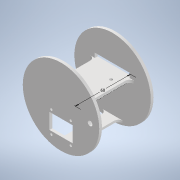
# Autodesk Inventor part: top2
Saved by Autodesk Inventor 2022 (Build 260153000, 153)
## iProperties
Created: 2025-06-18
Part Number: top2
Material: Типовые
Document SubType Name: Modeling
Designer: korsh624
Density: 1 g/cm^3
Appearance: По умолчанию
Author: korsh624
Autodesk Inventor part; units mm, degrees
ref_plane "YZ Plane" through (0, 0, 0) normal (1, 0, 0) x (0, 1, 0)
ref_plane "XZ Plane" through (0, 0, 0) normal (0, 1, 0) x (-1, 0, 0)
ref_plane "XY Plane" through (0, 0, 0) normal (0, 0, 1) x (1, 0, 0)
sketch "Эскиз3" plane through (0, 0, 0) normal (0, 0, 1) x (1, 0, 0)
  circle A0 centre (0, 0) radius 41.5
  line L0 (12.5, -11.0597) -> (-12.5, -11.0597) projected
  line L1 (-12.5, -11.0597) -> (-12.5, -28.0597) projected
  line L2 (-12.5, -11.0597) -> (12.5, -11.0597)
  line L3 (12.5, -11.0597) -> (12.5, -28.0597)
  line L4 (12.5, -28.0597) -> (-12.5, -28.0597)
  line L5 (-12.5, -28.0597) -> (-12.5, -11.0597)
  dimension "d9" = 83
  dimension "d10" = 25
  dimension "d11" = 17
  dimension "d13" = 25
  dimension "d14" = 17
  dimension "d15" = 12.5
  constraints: 8 end point, 2 parallel, 1 centre point, 1 coincident, 1 horizontal, 1 perpendicular
  measures "d9" diameter of A0
  measures "d10" distance of L0.start L0.end
  measures "d11" distance of L0.end L1.end
  measures "d13" distance of L2.start L2.end
  measures "d14" distance of L2.end L3.end
  measures "d15" distance from line of point (0, 0) L5
extrude "Выдавливание3" add sketch "Эскиз3" along normal blind 3
sketch "Эскиз4" plane through (0, 0, 3) normal (0, 0, 1) x (1, 0, 0)
  arc A0 (5.7629, -8.6636) -> (-4.709, -8.7124) centre (0.4132, 15.7598) ccw
  circle A1 centre (0.4132, 15.7598) radius 1.5338
  point P0 (0, 0)
  constraints: 2 centre point, 2 point on circle, 1 coincident, 4 other
extrude "Выдавливание4" cut sketch "Эскиз4" against normal blind 3
sketch "Эскиз5" plane through (0, 0, 3) normal (0, 0, 1) x (1, 0, 0)
  line L0 (28.2027, -2.4247) -> (31.5626, 4.2424) projected
  circle A0 centre (31.5626, 0.0623) radius 2.5
  point P0 (0, 0)
  dimension "d20" = 5
  constraints: 1 centre point
  measures "d20" diameter of A0
extrude "Выдавливание5" cut sketch "Эскиз5" against normal blind 3
sketch "Эскиз6" plane through (0, 0, 3) normal (0, 0, 1) x (1, 0, 0)
  circle A0 centre (0.4132, 15.7598) radius 1.5338 projected
  point P0 (0, 0)
extrude "Выдавливание6" add sketch "Эскиз6" against normal blind 3
sketch "Эскиз7" plane through (0, 0, 3) normal (0, 0, 1) x (1, 0, 0)
  circle A0 centre (10.5, -7.8097) radius 1.25 projected
  circle A1 centre (-10.5, -7.8097) radius 1.25 projected
  circle A2 centre (-10.5, -31.3097) radius 1.25 projected
  circle A3 centre (10.5, -31.3097) radius 1.25 projected
  point P0 (0, 0)
extrude "Выдавливание7" cut sketch "Эскиз7" against normal blind 3
sketch "Эскиз8" plane through (0, 0, 0) normal (0, 0, -1) x (-1, 0, 0)
  line L0 (-18.7254, 8.2596) -> (19.2746, 8.2596) projected
  line L1 (-18.7254, 8.2596) -> (19.2746, 8.2596)
  line L2 (19.2746, 8.2596) -> (19.2746, 5.2596)
  line L3 (19.2746, 5.2596) -> (-18.7254, 5.2596)
  line L4 (-18.7254, 5.2596) -> (-18.7254, 8.2596)
  point P0 (0, 0)
  dimension "d27" = 3
  constraints: 8 end point, 2 parallel, 1 horizontal, 1 perpendicular
  measures "d27" distance of L1.end L2.end
extrude "Выдавливание8" add sketch "Эскиз8" along normal blind 56
sketch "Эскиз9" plane through (-19.2746, 8.2596, 0) normal (0, 1, 0) x (1, 0, 0)
  circle A0 centre (29, 41.5) radius 1.6 projected
  circle A1 centre (22.71, 4.4641) radius 1.6 projected
  point P0 (19.2746, 0)
extrude "Выдавливание9" cut sketch "Эскиз9" against normal blind 56
sketch "Эскиз10" plane through (-19.2746, 5.2596, 0) normal (0, -1, 0) x (1, 0, 0)
  line L0 (0, 0) -> (38, 0) projected
  line L1 (38, 0) -> (38, -60) construction
  point P0 (19.2746, 0)
  dimension "d32" = 60
  constraints: 2 end point, 1 vertical
  measures "d32" distance of L0.end L1.end
sketch "Эскиз11" plane through (0, 0, -56) normal (0, 0, -1) x (-1, 0, 0)
  circle A0 centre (0, 0) radius 41.5 projected
  line L0 (-18.7254, 5.2596) -> (19.2746, 5.2596) projected
  line L1 (19.2746, 5.2596) -> (19.2746, 8.2596) projected
  line L2 (19.2746, 8.2596) -> (-18.7254, 8.2596) projected
  line L3 (-18.7254, 8.2596) -> (-18.7254, 5.2596) projected
  line L4 (-18.7254, 5.2596) -> (-18.7254, 8.2596) projected
  line L5 (-18.7254, 8.2596) -> (19.2746, 8.2596)
  line L6 (19.2746, 8.2596) -> (19.2746, 13.2596)
  line L7 (19.2746, 13.2596) -> (-18.7254, 13.2596)
  line L8 (-18.7254, 13.2596) -> (-18.7254, 8.2596)
  dimension "d33" = 5
  constraints: 8 end point, 2 parallel, 1 horizontal, 1 perpendicular
  measures "d33" distance of L6.end L5.end
extrude "Выдавливание10" add sketch "Эскиз11" against normal blind 3
sketch "Эскиз12" plane through (0, 0, 0) normal (0, 0, -1) x (-1, 0, 0)
  circle A0 centre (0, 0) radius 41.5 projected
  line L0 (-6.5, -33.0597) -> (-6.5, -30.5597) projected
  line L1 (6.5, -33.0597) -> (6.5, -30.5597) projected
  line L2 (-6.5, -35.5314) -> (6.5, -35.5314)
  line L3 (6.5, -35.5314) -> (6.5, -37.9075)
  line L4 (6.5, -37.9075) -> (-6.5, -37.9075)
  line L5 (-6.5, -37.9075) -> (-6.5, -35.5314)
  constraints: 8 end point, 2 parallel, 1 horizontal, 1 perpendicular
extrude "Выдавливание11" add sketch "Эскиз12" along normal blind 54.75 contours L2 L3 L4 L5
fillet "Сопряжение1" radius 5 8 edges at (-19.2746, 6.7596, 0) (18.7254, 6.7596, 0) (6.5, -36.7195, 0) (-6.5, -36.7195, 0) (-6.5, -36.7195, -53) (-19.2746, 6.7596, -53) (6.5, -36.7195, -53) (18.7254, 6.7596, -53)
equation "\"d13\" = d10"
equation "\"d14\" = d11"
equation "\"d15\" = 0.5 * d13"
